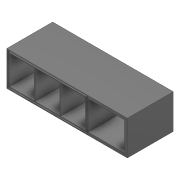
# Autodesk Inventor part: 3Eier_größer
Saved by Autodesk Inventor 2020 (Build 240168000, 168)
## iProperties
Created: 2021-09-03
Part Number: 3Eier_größer
Material: Acetalharz, Schwarz
Document SubType Name: Modeling
Designer: Julian Uhl
Density: 1.425 g/cm^3
Appearance: Glatt - Schwarz
Author: Julian Uhl
Autodesk Inventor part; units mm, degrees
ref_plane "YZ Plane" through (0, 0, 0) normal (1, 0, 0) x (0, 1, 0)
ref_plane "XZ Plane" through (0, 0, 0) normal (0, 1, 0) x (-1, 0, 0)
ref_plane "XY Plane" through (0, 0, 0) normal (0, 0, 1) x (1, 0, 0)
sketch "Skizze1" plane through (0, 0, 0) normal (0, 0, 1) x (1, 0, 0)
  line L0 (-99.7629, 0) -> (488.2371, 0) projected
  line L1 (0, -39.9766) -> (0, 128.0234) projected
  line L2 (-5.7629, 94.0234) -> (394.2371, 94.0234)
  line L3 (394.2371, 94.0234) -> (394.2371, -5.9766)
  line L4 (394.2371, -5.9766) -> (-5.7629, -5.9766)
  line L5 (-5.7629, -5.9766) -> (-5.7629, 94.0234)
  line L6 (80.2371, 94.0234) -> (80.2371, -5.9766)
  line L7 (83.2371, -5.9766) -> (83.2371, 94.0234)
  line L8 (169.2371, 94.0234) -> (169.2371, -5.9766)
  line L9 (172.2371, -5.9766) -> (172.2371, 94.0234)
  line L10 (258.2371, 94.0234) -> (258.2371, -5.9766)
  line L11 (268.2371, -5.9766) -> (268.2371, 94.0234)
  line L12 (-15.7629, 104.0234) -> (404.2371, 104.0234)
  line L13 (404.2371, 104.0234) -> (404.2371, -15.9766)
  line L14 (404.2371, -15.9766) -> (-15.7629, -15.9766)
  line L15 (-15.7629, -15.9766) -> (-15.7629, 104.0234)
  point P0 (0, 0)
  point P1 (274.2371, 94.0234)
  point P2 (180.9371, 94.0234)
  point P3 (87.6371, 94.0234)
  dimension "d0" = 100
  dimension "d1" = 400
  dimension "d2" = 120
  dimension "d11" = 10
  dimension "d12" = 10
  dimension "d13" = 10
  dimension "d14" = 10
  dimension "d20" = 86
  dimension "d21" = 86
  dimension "d22" = 86
  dimension "d23" = 3
  dimension "d24" = 3
  dimension "d25" = 10
  constraints: 26 end point, 6 point on line, 4 vertical, 3 parallel, 3 perpendicular, 2 horizontal, 12 other
  measures "d1" distance between parallel lines of L3 L5
  measures "d2" distance from line of L3 point (274.237, 94.023)
  measures "d11" distance between parallel lines of L13 L3
  measures "d12" distance between parallel lines of L14 L4
  measures "d14" distance between parallel lines of L5 L15
  measures "d20" distance between parallel lines of L6 L5
  measures "d21" distance between parallel lines of L8 L7
  measures "d22" distance between parallel lines of L10 L9
  measures "d23" distance between parallel lines of L7 L6
  measures "d24" distance between parallel lines of L9 L8
  measures "d25" distance between parallel lines of L11 L10
extrude "Extrusion1" add sketch "Skizze1" along normal blind 150 contours L15 L12 L1 L2 L5 L0 | L0 L5 L4 L1 L14 L15 | L1 L4 L3 L0 L13 L14 | L12 L13 L0 L3 L2 L1 | L6 L2 L7 L0 | L0 L7 L4 L6 | L8 L2 L9 L0 | L0 L9 L4 L8 | L11 L4 L10 L0 | L0 L10 L2 L11
sketch "Skizze2" plane through (0, 0, 0) normal (0, 0, -1) x (-1, 0, 0)
  line L0 (15.7629, -15.9766) -> (-404.2371, -15.9766) projected
  line L1 (-404.2371, -15.9766) -> (-404.2371, 104.0234) projected
  line L2 (15.7629, -15.9766) -> (-404.2371, -15.9766)
  line L3 (-404.2371, -15.9766) -> (-404.2371, 104.0234)
  line L4 (-404.2371, 104.0234) -> (15.7629, 104.0234)
  line L5 (15.7629, 104.0234) -> (15.7629, -15.9766)
  point P0 (0, 0)
  constraints: 8 end point, 2 parallel, 1 horizontal, 1 perpendicular
extrude "Extrusion2" add sketch "Skizze2" along normal blind 10
sketch "Skizze3" plane through (80.2371, -5.9766, 150) normal (-1, 0, 0) x (0, 0, 1)
  point P0 (-150, 5.9766)
sketch "Skizze4" plane through (0, 0, 150) normal (0, 0, 1) x (1, 0, 0)
  line L0 (-13.2629, 101.5234) -> (265.7371, 101.5234)
  line L1 (265.7371, 101.5234) -> (265.7371, 96.5234)
  line L2 (265.7371, 96.5234) -> (-13.2629, 96.5234)
  line L3 (-13.2629, 96.5234) -> (-13.2629, 101.5234)
  line L4 (260.7371, 96.5234) -> (265.7371, 96.5234)
  line L5 (265.7371, 96.5234) -> (265.7371, -13.6946)
  line L6 (265.7371, -13.6946) -> (260.7371, -13.6946)
  line L7 (260.7371, -13.6946) -> (260.7371, 96.5234)
  line L8 (260.7371, -8.4766) -> (-13.2629, -8.4766)
  line L9 (-13.2629, -8.4766) -> (-13.2629, -13.4766)
  line L10 (-13.2629, -13.4766) -> (260.7371, -13.4766)
  line L11 (260.7371, -13.4766) -> (260.7371, -8.4766)
  line L12 (-13.2629, -8.4766) -> (-8.2629, -8.4766)
  line L13 (-8.2629, -8.4766) -> (-8.2629, 96.5234)
  line L14 (-8.2629, 96.5234) -> (-13.2629, 96.5234)
  line L15 (-13.2629, 96.5234) -> (-13.2629, -8.4766)
  line L16 (404.2371, 104.0234) -> (-15.7629, 104.0234) projected
  line L17 (-5.7629, 94.0234) -> (80.2371, 94.0234) projected
  line L18 (-5.7629, -5.9766) -> (-5.7629, 94.0234) projected
  line L19 (-15.7629, 104.0234) -> (-15.7629, -15.9766) projected
  line L20 (80.2371, -5.9766) -> (-5.7629, -5.9766) projected
  line L21 (-15.7629, -15.9766) -> (404.2371, -15.9766) projected
  line L22 (258.2371, 94.0234) -> (258.2371, -5.9766) projected
  line L23 (268.2371, -5.9766) -> (268.2371, 94.0234) projected
  point P0 (0, 0)
  point P1 (400.2371, 104.0234)
  point P2 (-11.7629, 104.0234)
  point P3 (-15.7629, 100.0234)
  point P4 (-15.7629, -11.9766)
  point P5 (-11.7629, -15.9766)
  point P6 (400.2371, -15.9766)
  point P7 (-13.2629, 96.5234)
  dimension "d26" = 2.5
  dimension "d27" = 2.5
  dimension "d28" = 2.5
  dimension "d29" = 2.5
  dimension "d30" = 2.5
  dimension "d31" = 2.5
  dimension "d32" = 2.5
  dimension "d33" = 2.5
  dimension "d34" = 2.5
  constraints: 32 end point, 8 parallel, 4 horizontal, 4 perpendicular, 4 point on line
  measures "d26" distance between parallel lines of L16 L0
  measures "d27" distance between parallel lines of L17 L2
  measures "d28" distance between parallel lines of L18 L13
  measures "d29" distance between parallel lines of L19 L15
  measures "d30" distance between parallel lines of L19 L3
  measures "d31" distance between parallel lines of L20 L8
  measures "d32" distance between parallel lines of L21 L10
  measures "d33" distance between parallel lines of L22 L7
  measures "d34" distance between parallel lines of L23 L5
extrude "Extrusion3" cut sketch "Skizze4" against normal blind 5 contours L0 L1 L2 L3 | L2 L13 L8 L15 | L5 L6 L7 L2 | L8 L7 L10 L9
